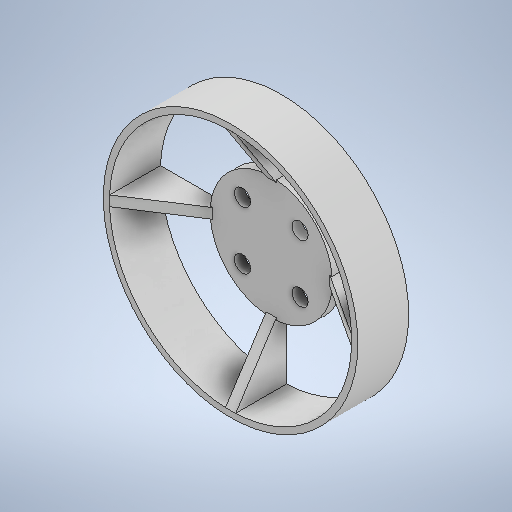
# Autodesk Inventor part: Wheel-D50A
Saved by Autodesk Inventor 2025.3 (Build 293356000, 356)
## iProperties
Created: 2025-07-18
Part Number: Wheel-D50A
Material: 一般
Document SubType Name: Modeling
Designer: yamashita1
Density: 1 g/cm^3
Appearance: 既定
Author: yamashita1
Autodesk Inventor part; units mm, degrees
ref_plane "YZ Plane" through (0, 0, 0) normal (1, 0, 0) x (0, 1, 0)
ref_plane "XZ Plane" through (0, 0, 0) normal (0, 1, 0) x (-1, 0, 0)
ref_plane "XY Plane" through (0, 0, 0) normal (0, 0, 1) x (1, 0, 0)
sketch "スケッチ1" plane through (0, 0, 0) normal (0, 0, 1) x (1, 0, 0)
  circle A0 centre (0, 0) radius 12
  dimension "d0" = 24
  constraints: 1 centre point, 1 coincident
  measures "d0" diameter of A0
extrude "ハブ" add sketch "スケッチ1" along normal blind 2
sketch "スケッチ2" plane through (0, 0, 0) normal (0, 0, 1) x (1, 0, 0)
  circle A0 centre (0, 0) radius 25
  circle A1 centre (0, 0) radius 23.8
  dimension "d3" = 50
  dimension "d4" = 1.2
  constraints: 2 centre point, 2 coincident
  measures "d3" diameter of A0
  measures "d4" radial gap between concentric circles of A0 A1
extrude "リム" add sketch "スケッチ2" along normal blind 10
sketch "スケッチ5" plane through (0, 0, 0) normal (1, 0, 0) x (0, 1, 0)
  line L0 (23.8, 10) -> (23.8, 0) projected
  line L1 (23.8, 10) -> (23.8, 0)
  line L2 (23.8, 0) -> (11.5, 0)
  line L3 (25, 0) -> (-25, 0) projected
  line L4 (11.5, 0) -> (11.5, 2)
  line L5 (11.5, 2) -> (23.8, 10)
  line L6 (12, 2) -> (-12, 2) projected
  point P0 (0, 0)
  point P1 (0, 0)
  dimension "d10" = 11.5
  constraints: 8 end point, 4 point on line, 1 midpoint, 1 vertical
  measures "d10" distance from line of point (0, 0) L4
extrude "スポーク" add sketch "スケッチ5" along normal mid plane 2
pattern_circular "円形状パターン1" count 4 over 360 about axis through (0, 0, -10) along (0, 0, 1) of "スポーク"
sketch "スケッチ6" plane through (0, 0, 2) normal (0, 0, 1) x (1, 0, 0)
  circle A0 centre (0, 0) radius 8 construction
  line L0 (-13.4189, -13.4189) -> (13.4189, 13.4189) construction
  line L1 (-15.0493, 15.0493) -> (15.0493, -15.0493) construction
  line L2 (-16.6434, 0) -> (16.6434, 0) construction
  point P0 (5.6569, 5.6569)
  point P1 (-5.6569, 5.6569)
  point P2 (-5.6569, -5.6569)
  point P3 (5.6569, -5.6569)
  dimension "d16" = 16
  dimension "d17" = 45
  dimension "d18" = 45
  constraints: 6 end point, 4 point on circle, 4 point on line, 3 midpoint, 2 coincident, 1 centre point, 1 horizontal
  measures "d16" diameter of A0
  measures "d17" angle of L0 L2
  measures "d18" angle of L2 L1
hole "穴1" at (5.6569, 5.6569, 2) at (-5.6569, 5.6569, 2) at (-5.6569, -5.6569, 2) at (5.6569, -5.6569, 2) direction (0, 0, -1) diameter 3.2 end through all
equation "\"d18\" = d17"
